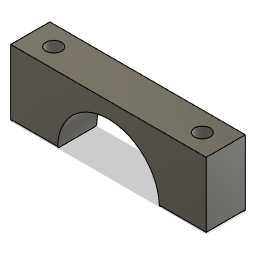
Lock (Autodesk Fusion 360 design; units mm, degrees)
Autodesk Fusion 360 part; units mm, degrees
sketch "Sketch1" plane through (0, 0, 0) normal (0, 0, 1) x (1, 0, 0)
  line L0 (25, 0) -> (25, 8.5)
  line L1 (25, 8.5) -> (0, 8.5)
  line L2 (0, 8.5) -> (0, 0)
  arc A0 (19, 0) -> (6, 0) centre (12.5, 0) ccw
  line L3 (0, 0) -> (6, 0)
  line L4 (19, 0) -> (25, 0)
  dimension "d1" = 25
  dimension "d2" = 8.5
  dimension "d3" = 13
  constraint horizontal L3
  constraint vertical L0
  constraint horizontal L1
  constraint vertical L2
  constraint coincident L2.end L3.start
  constraint coincident A0.start L3
  constraint collinear L3 L4
  constraint coincident A0.centre L3
  measures "d1" distance of L2.end L0.start
  measures "d2" distance of L2.end L1.end
  measures "d3" diameter of A0
extrude "Extrude1" add sketch "Sketch1" along normal blind 5
sketch "Sketch2" plane through (0, 8.5, 0) normal (0, 1, 0) x (-1, 0, 0)
  line L0 (-25, 0) -> (0, 0)
  line L1 (0, 0) -> (0, 5)
  line L2 (0, 5) -> (-25, 5)
  line L3 (-25, 5) -> (-25, 0)
  line L4 (-19, 0) -> (-19, 5)
  line L5 (-6, 0) -> (-6, 5)
  line L6 (0, 5) -> (-6, 0) construction
  line L7 (-12.5, 0) -> (-12.5, 5)
  circle A0 centre (-3, 2.5) radius 1
  circle A1 centre (-22, 2.5) radius 1
  dimension "d6" = 2
  constraint coincident L1.end L2.start
  constraint coincident L5.start L6.end
  constraint midpoint L0 L7.start
  constraint midpoint L2 L7.end
  constraint midpoint L6 A0.centre
  constraint symmetric L7 A0 A1
  measures "d6" diameter of A0
extrude "Extrude2" cut sketch "Sketch2" against normal through all contours A0 | A1
fillet "Fillet1" radius 0.2 6 edges at (0, 0, 2.5) (3, 0, 0) (3, 0, 5) (22, 0, 5) (25, 0, 2.5) (22, 0, 0)
